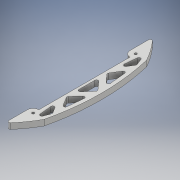
# Autodesk Inventor part: ガイド横v1
Saved by Autodesk Inventor 2018.3 (Build 223284000, 284)
## iProperties
Created: 2019-02-14
Part Number: ガイド横v1
Material: 一般
Document SubType Name: Modeling
Designer: shun2
Density: 1 g/cm^3
Appearance: 既定
Author: shun2
Autodesk Inventor part; units mm, degrees
ref_plane "YZ Plane" through (0, 0, 0) normal (1, 0, 0) x (0, 1, 0)
ref_plane "XZ Plane" through (0, 0, 0) normal (0, 1, 0) x (-1, 0, 0)
ref_plane "XY Plane" through (0, 0, 0) normal (0, 0, 1) x (1, 0, 0)
sketch "スケッチ1" plane through (0, 0, 0) normal (0, 0, 1) x (1, 0, 0)
  circle A0 centre (7, 27.638) radius 1.5
  circle A1 centre (7, 152.362) radius 1.5
  arc A2 (20.2574, 27.638) -> (20.2574, 152.362) centre (-242.442, 90) ccw
  arc A3 (0, 0) -> (20.2574, 27.638) centre (-93.8083, 90) ccw
  arc A4 (20.2574, 152.362) -> (0, 180) centre (-93.8083, 90) ccw
  arc A5 (0, 152.362) -> (7, 145.362) centre (7, 152.362) ccw
  arc A6 (7, 34.638) -> (0, 27.638) centre (7, 27.638) ccw
  line L0 (7, 34.638) -> (7, 145.362)
  line L1 (0, 180) -> (0, 152.362)
  line L2 (0, 27.638) -> (0, 0)
  point P0 (7, 20.638)
  point P1 (7, 159.362)
  dimension "d2" = 3
  dimension "d11" = 27.638
  dimension "d12" = 270
  constraints: 10 point on circle, 7 centre point, 6 end point, 3 vertical, 2 coincident, 2 point on line
  measures "d2" diameter of A0
  measures "d11" vertical distance of L2.end A0.centre
  measures "d12" radius of A2
extrude "押し出し1" add sketch "スケッチ1" along normal blind 7
sketch "スケッチ2" plane through (0, 0, 7) normal (0, 0, 1) x (1, 0, 0)
  line L0 (10, 80.2837) -> (10, 99.7163)
  line L1 (13.4987, 101.0407) -> (22.0846, 91.3243)
  line L2 (22.0846, 88.6757) -> (13.4987, 78.9593)
  line L3 (19.2111, 75.7008) -> (11.0046, 66.6519)
  line L4 (10.7784, 64.2673) -> (17.1291, 53.8503)
  line L5 (20.8277, 54.7016) -> (22.6836, 74.1675)
  line L6 (14.4979, 46.7358) -> (18.8075, 39.7711)
  line L7 (18.979, 38.0154) -> (16.0642, 30.2561)
  line L8 (12.2009, 30.7708) -> (10.8061, 45.4948)
  arc A0 (18.979, 38.0154) -> (18.8075, 39.7711) centre (17.1068, 38.7188) ccw
  arc A1 (11.0046, 66.6519) -> (10.7784, 64.2673) centre (12.4861, 65.3083) ccw
  arc A2 (22.0846, 88.6757) -> (22.0846, 91.3243) centre (20.5859, 90) ccw
  arc A3 (12.2009, 30.7708) -> (16.0642, 30.2561) centre (14.192, 30.9595) ccw
  arc A4 (14.4979, 46.7358) -> (10.8061, 45.4948) centre (12.7972, 45.6834) ccw
  arc A5 (17.1291, 53.8503) -> (20.8277, 54.7016) centre (18.8368, 54.8914) ccw
  arc A6 (22.6836, 74.1675) -> (19.2111, 75.7008) centre (20.6926, 74.3573) ccw
  arc A7 (10, 80.2837) -> (13.4987, 78.9593) centre (12, 80.2837) ccw
  arc A8 (13.4987, 101.0407) -> (10, 99.7163) centre (12, 99.7163) ccw
  line L9 (19.2111, 104.2992) -> (11.0046, 113.3481)
  line L10 (10.7784, 115.7327) -> (17.1291, 126.1497)
  line L11 (20.8277, 125.2984) -> (22.6836, 105.8325)
  line L12 (14.4979, 133.2642) -> (18.8075, 140.2289)
  line L13 (18.979, 141.9846) -> (16.0642, 149.7439)
  line L14 (12.2009, 149.2292) -> (10.8061, 134.5052)
  arc A9 (18.8075, 140.2289) -> (18.979, 141.9846) centre (17.1068, 141.2812) ccw
  arc A10 (10.7784, 115.7327) -> (11.0046, 113.3481) centre (12.4861, 114.6917) ccw
  arc A11 (16.0642, 149.7439) -> (12.2009, 149.2292) centre (14.192, 149.0405) ccw
  arc A12 (10.8061, 134.5052) -> (14.4979, 133.2642) centre (12.7972, 134.3166) ccw
  arc A13 (20.8277, 125.2984) -> (17.1291, 126.1497) centre (18.8368, 125.1086) ccw
  arc A14 (19.2111, 104.2992) -> (22.6836, 105.8325) centre (20.6926, 105.6427) ccw
  point P0 (0, 0)
  point P1 (10, 75)
  point P2 (10, 105)
  dimension "d17" = 30
  dimension "d18" = 2
  constraints: 30 end point, 30 point on circle, 18 tangent, 15 centre point, 8 equal radius, 4 point on line, 1 vertical
  measures "d17" distance of point (10, 75) point (10, 105)
  measures "d18" radius of A0
extrude "押し出し2" cut sketch "スケッチ2" against normal blind 7
fillet "フィレット1" radius 2 2 edges at (0, 180, 3.5) (0, 0, 3.5)
